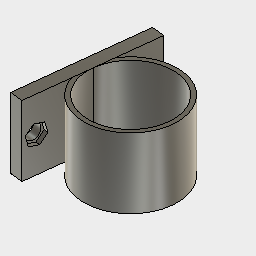
bart lm10uu bed bearing mount v2 (Autodesk Fusion 360 design; units mm, degrees)
Autodesk Fusion 360 part; units mm, degrees
sketch "Sketch1" plane through (0, 0, 0) normal (0, 0, 1) x (1, 0, 0)
  circle A0 centre (0, 0) radius 10
  circle A1 centre (0, 0) radius 11
  dimension "d1" = 20
  dimension "d2" = 22
  measures "d1" diameter of A0
  measures "d2" diameter of A1
extrude "Extrude1" add sketch "Sketch1" along normal blind 16.5 makes body 1
ref_plane "WorkPlane3" through (-9.935, 1.1383, 16.5773) normal (0.9935, -0.113828, 0) x (-0.113828, -0.9935, 0)
sketch "Sketch3" plane through (-9.935, 1.1383, 16.5773) normal (0.9935, -0.113828, 0) x (-0.113828, -0.9935, 0)
  line L0 (-20.2183, -12.4227) -> (20.0583, -12.4227)
  line L1 (20.0583, -12.4227) -> (20.0583, 16.5773)
  line L2 (20.0583, 16.5773) -> (-20.2183, 16.5773)
  line L3 (-20.2183, 16.5773) -> (-20.2183, -12.4227)
  constraint horizontal L0
  constraint vertical L1
  constraint horizontal L2
  constraint vertical L3
sketch "Sketch4" plane through (0, 0, 16.5) normal (0, 0, 1) x (-1, 0, 0)
  circle A0 centre (0, 0) radius 10
  circle A1 centre (0, 0) radius 11
  circle A2 centre (0, 0) radius 11
  line L0 (9.4199, -5.6802) -> (10.4907, 3.3083)
  arc A3 (9.4199, -5.6802) -> (10.4907, 3.3083) centre (0, 0) ccw
  constraint coincident A1
  constraint concentric A2 A3
extrude "Extrude3" cut sketch "Sketch4" against normal blind 29 contours A1 A2 L0 A3 bodies 1
extrude "Extrude4" cut sketch "Sketch3" against normal blind 3 bodies 1
sketch "Sketch5" plane through (-9.935, 1.1383, 0) normal (-0.9935, 0.113828, 0) x (-0.113828, -0.9935, 0)
  line L0 (0, 0) -> (4.5826, 0)
  line L1 (4.5826, 16.5) -> (0, 16.5)
  line L2 (0, 16.5) -> (-4.5826, 16.5)
  line L3 (-4.5826, 0) -> (0, 0)
  line L4 (-15.0065, 16.5006) -> (15.2015, 16.5006)
  line L5 (15.2015, 16.5006) -> (15.2015, -0.061)
  line L6 (15.2015, -0.061) -> (-15.0065, -0.061)
  line L7 (-15.0065, -0.061) -> (-15.0065, 16.5006)
  line L8 (0, 0) -> (0, 16.5)
  line L9 (0, 16.5) -> (0, 0)
  constraint horizontal L4
  constraint vertical L5
  constraint horizontal L6
  constraint vertical L7
extrude "Extrude5" add sketch "Sketch5" along normal blind 3 separate body makes body 2
sketch "Sketch6" plane through (-12.9155, 1.4798, 0) normal (-0.9935, 0.113828, 0) x (-0.113828, -0.9935, 0)
  line L0 (-15.0065, -0.061) -> (15.2015, -0.061)
  line L1 (15.2015, -0.061) -> (15.2015, 16.5006)
  line L2 (15.2015, 16.5006) -> (-15.0065, 16.5006)
  line L3 (-15.0065, 16.5006) -> (-15.0065, -0.061)
  line L4 (-22.3492, 8.2198) -> (26.4176, 8.2198)
  line L5 (-12.067, 16.5006) -> (-12.067, -5.8744)
  line L6 (12.048, 16.5006) -> (12.048, -2.9739)
  constraint perpendicular L3 L4
  constraint coincident L2
  constraint perpendicular L2 L5
  constraint perpendicular L0 L6
sketch "Sketch7" plane through (0, 0, 0) normal (0, 0, -1) x (1, 0, 0)
  line L0 (-10.4566, 3.4145) -> (-9.935, -1.1383)
  circle A0 centre (0, 0) radius 10
  line L1 (-9.935, -1.1383) -> (-9.4134, -5.6911)
  arc A1 (-9.4134, -5.6911) -> (-10.4566, 3.4145) centre (0, 0) ccw
  circle A2 centre (0, 0) radius 9.0342
  constraint concentric A0 A2
extrude "Extrude6" add sketch "Sketch7" against normal blind 2 separate body contours A0 makes body 3
sketch "Sketch8" plane through (-12.9155, 1.4798, 0) normal (-0.9935, 0.113828, 0) x (-0.113828, -0.9935, 0)
  line L0 (-15.0065, -0.061) -> (15.2015, -0.061)
  line L1 (15.2015, -0.061) -> (15.2015, 16.5006)
  line L2 (15.2015, 16.5006) -> (-15.0065, 16.5006)
  line L3 (-15.0065, 16.5006) -> (-15.0065, -0.061)
  line L4 (-12.067, 16.5006) -> (-12.067, -5.8744)
  line L5 (-22.3492, 8.2198) -> (26.4176, 8.2198)
  constraint coincident L4
  constraint coincident L5
hole "Hole1" at (-11.5419, 13.4684, 8.2198) at (-14.2911, -10.5267, 8.2198) direction (0.9935, -0.113828, 0) diameter 3.5 depth 4 tip angle 118 bodies 2
sketch "Sketch9" plane through (-9.935, 1.1383, 0) normal (0.9935, -0.113828, 0) x (0.113828, 0.9935, 0)
  circle A0 centre (12.067, 8.2198) radius 1.75
  circle A1 centre (-12.085, 8.2198) radius 1.75
  line L0 (-15.2015, -0.061) -> (15.0065, -0.061)
  line L1 (15.0065, -0.061) -> (15.0065, 16.5006)
  line L2 (15.0065, 16.5006) -> (-15.2015, 16.5006)
  line L3 (-15.2015, 16.5006) -> (-15.2015, -0.061)
  line L4 (-14.5038, 8.8445) -> (-13.8354, 6.4375)
  line L5 (-13.8354, 6.4375) -> (-11.4167, 5.8127)
  line L6 (-11.4167, 5.8127) -> (-9.6663, 7.5951)
  line L7 (-9.6663, 7.5951) -> (-10.3346, 10.0021)
  line L8 (-10.3346, 10.0021) -> (-12.7534, 10.6268)
  line L9 (-12.7534, 10.6268) -> (-14.5038, 8.8445)
extrude "Extrude7" cut sketch "Sketch9" against normal blind 1 contours L4 L5 L6 L7 L8 L9 bodies 2
sketch "Sketch10" plane through (-9.935, 1.1383, 0) normal (0.9935, -0.113828, 0) x (0.113828, 0.9935, 0)
  line L0 (-13.8354, 6.4375) -> (-14.5038, 8.8445)
  line L1 (-14.5038, 8.8445) -> (-12.7534, 10.6268)
  line L2 (-12.7534, 10.6268) -> (-10.3346, 10.0021)
  line L3 (-10.3346, 10.0021) -> (-9.6663, 7.5951)
  line L4 (-9.6663, 7.5951) -> (-11.4167, 5.8127)
  line L5 (-11.4167, 5.8127) -> (-13.8354, 6.4375)
  circle A0 centre (12.067, 8.2198) radius 1.75
  line L6 (-15.2015, -0.061) -> (15.0065, -0.061)
  line L7 (15.0065, -0.061) -> (15.0065, 16.5006)
  line L8 (15.0065, 16.5006) -> (-15.2015, 16.5006)
  line L9 (-15.2015, 16.5006) -> (-15.2015, -0.061)
  line L10 (14.284, 6.9762) -> (14.2525, 9.518)
  line L11 (14.2525, 9.518) -> (12.0355, 10.7616)
  line L12 (12.0355, 10.7616) -> (9.85, 9.4634)
  line L13 (9.85, 9.4634) -> (9.8816, 6.9216)
  line L14 (9.8816, 6.9216) -> (12.0985, 5.678)
  line L15 (12.0985, 5.678) -> (14.284, 6.9762)
extrude "Extrude8" cut sketch "Sketch10" against normal blind 1 contours L10 L11 L12 L13 L14 L15 bodies 2
sketch "Sketch2" plane through (10.6005, 2.9377, 18.9846) normal (0.963678, 0.267068, 0) x (0.267068, -0.963678, 0)
  line L0 (15.126, -10.1835) -> (-14.9067, -10.1835)
  line L1 (-14.9067, -10.1835) -> (-14.9067, 19.0104)
  line L2 (-14.9067, 19.0104) -> (15.126, 19.0104)
  line L3 (15.126, 19.0104) -> (15.126, -10.1835)
  constraint horizontal L0
  constraint vertical L1
  constraint horizontal L2
  constraint vertical L3
extrude "Extrude2" [suppressed]
